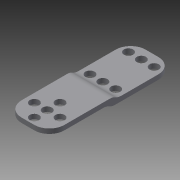
# Autodesk Inventor part: ArmToSide
Saved by Autodesk Inventor 2014 (Build 180170000, 170)
## iProperties
Created: 2014-03-07
Part Number: ArmToSide
Material: Générique
Document SubType Name: Modeling
Designer: Grégoire
Density: 1 g/cm^3
Appearance: Par défaut
Author: Grégoire
Autodesk Inventor part; units mm, degrees
ref_plane "YZ Plane" through (0, 0, 0) normal (1, 0, 0) x (0, 1, 0)
ref_plane "XZ Plane" through (0, 0, 0) normal (0, 1, 0) x (-1, 0, 0)
ref_plane "XY Plane" through (0, 0, 0) normal (0, 0, 1) x (1, 0, 0)
sketch "Esquisse5" plane through (0, 0, 0) normal (0, 0, 1) x (1, 0, 0)
  line L0 (0, 0) -> (20, 0)
  line L1 (20, 0) -> (20, 27)
  line L2 (20, 27) -> (0, 27)
  line L3 (0, 27) -> (0, 0)
  line L4 (10, 0) -> (10, 27) construction
  circle A0 centre (10, 3) radius 2.15
  circle A1 centre (10, 9) radius 2.15
  circle A2 centre (10, 15) radius 2.15
  line L5 (10, 9) -> (20, 9) construction
  circle A3 centre (16, 9) radius 2.15
  circle A4 centre (4, 9) radius 2.15
  circle A5 centre (10, 9) radius 2.15
  dimension "d61" = 20
  dimension "d62" = 27
  dimension "d63" = 3
  dimension "d64" = 4.3
  dimension "d67" = 6
  dimension "d74" = 6
  dimension "d77" = 6
  constraints: 12 end point, 6 centre point, 3 horizontal, 2 midpoint, 2 parallel, 2 perpendicular, 2 point on line, 1 vertical, 10 other
  measures "d61" distance of L0.start L0.end
  measures "d62" distance of L2.end L0.start
  measures "d63" distance from line of L0 A0.centre
  measures "d64" diameter of A0
  measures "d67" distance of A0.centre L5.start
  measures "d74" distance of L5.start A3.centre
  measures "d77" distance of L5.start A4.centre
extrude "Extrusion5" add sketch "Esquisse5" along normal blind 2.2
sketch "Esquisse6" plane through (0, 0, 2.2) normal (0, 0, 1) x (1, 0, 0)
  line L0 (0, 27) -> (20, 27)
  line L1 (20, 27) -> (20, 30)
  line L2 (20, 30) -> (0, 30)
  line L3 (0, 30) -> (0, 27)
  dimension "d82" = 3
  constraints: 8 end point, 2 parallel, 1 horizontal, 1 perpendicular
  measures "d82" distance of L2.end L0.start
extrude "Extrusion6" add sketch "Esquisse6" against normal blind 3.7
sketch "Esquisse7" plane through (0, 30, 2.2) normal (0, 1, 0) x (1, 0, 0)
  line L0 (20, 0) -> (20, 3.7) construction
  line L1 (0, 3.7) -> (20, 3.7)
  line L2 (20, 3.7) -> (20, 1.5)
  line L3 (20, 1.5) -> (0, 1.5)
  line L4 (0, 1.5) -> (0, 3.7)
  line L5 (20, 3.7) -> (0, 3.7) projected
  point P0 (0, 2.2)
  dimension "d85" = 2.2
  constraints: 8 end point, 2 parallel, 1 horizontal, 1 perpendicular, 1 point on line
  measures "d85" distance between parallel lines of L5 L3
extrude "Extrusion7" add sketch "Esquisse7" along normal blind 28
sketch "Esquisse8" plane through (0, 30, 0.7) normal (0, 0, 1) x (1, 0, 0)
  line L0 (20, 0) -> (0, 0) construction
  line L1 (20, 0) -> (20, 28) construction
  line L2 (0, 28) -> (20, 28) construction
  line L3 (10, 28) -> (10, 0) construction
  circle A0 centre (10, 23) radius 2.15
  line L4 (10, 23) -> (20, 23) construction
  circle A1 centre (16, 23) radius 2.15
  circle A2 centre (4, 23) radius 2.15
  circle A3 centre (10, 23) radius 2.15
  circle A4 centre (10, 5) radius 2.15
  circle A5 centre (16, 5) radius 2.15
  circle A6 centre (4, 5) radius 2.15
  point P0 (0, -30)
  dimension "d88" = 5
  dimension "d89" = 4.3
  dimension "d92" = 6
  dimension "d95" = 6
  dimension "d104" = 18
  constraints: 7 centre point, 4 end point, 2 horizontal, 2 midpoint, 2 point on line, 1 perpendicular, 1 vertical, 12 other
  measures "d88" distance from line of L2 L4.start
  measures "d89" diameter of A0
  measures "d92" distance of L4.start A1.centre
  measures "d95" distance of L4.start A2.centre
  measures "d104" distance of A2.centre A6.centre
extrude "Extrusion8" cut sketch "Esquisse8" against normal through all
fillet "Congé4" radius 7 4 edges at (0, 58, -0.4) (20, 58, -0.4) (0, 0, 1.1) (20, 0, 1.1)
fillet "Congé5" radius 5 4 edges at (10, 27, 0) (10, 27, -1.5) (10, 30, 2.2) (10, 30, 0.7)
equation "\"d64\" = Holes"
equation "\"d80\" = Depth"
equation "\"d85\" = Depth"
equation "\"d89\" = Holes"
equation "\"d100\" = Rounding"
equation "\"Depth\" = 2.2"
equation "\"Holes\" = 4.3"
equation "\"Height\" = 0"
equation "\"Rounding\" = 7"
